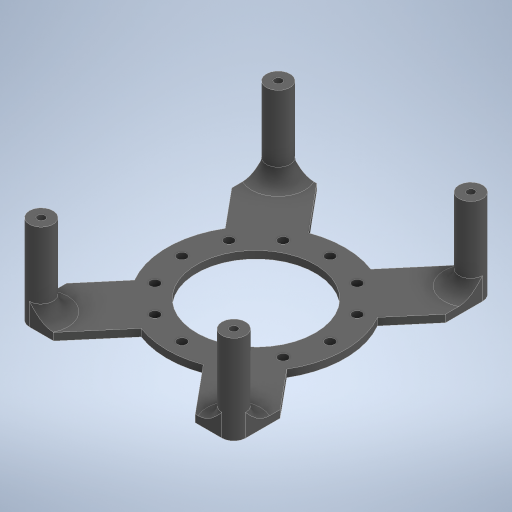
# Autodesk Inventor part: board_base_connect
Saved by Autodesk Inventor 2024.1 (Build 281209000, 209)
## iProperties
Created: 2024-08-02
Part Number: board_base_connect
Material: 一般
Document SubType Name: Modeling
Designer: hibik
Density: 1 g/cm^3
Appearance: 既定
Author: hibik
Autodesk Inventor part; units mm, degrees
ref_plane "YZ Plane" through (0, 0, 0) normal (1, 0, 0) x (0, 1, 0)
ref_plane "XZ Plane" through (0, 0, 0) normal (0, 1, 0) x (-1, 0, 0)
ref_plane "XY Plane" through (0, 0, 0) normal (0, 0, 1) x (1, 0, 0)
sketch "スケッチ1" plane through (0, 0, 0) normal (0, 1, 0) x (-1, 0, 0)
  line L0 (-32.5, -40) -> (32.5, -40) construction
  line L1 (32.5, -40) -> (32.5, 40) construction
  line L2 (32.5, 40) -> (-32.5, 40) construction
  line L3 (-32.5, 40) -> (-32.5, -40) construction
  line L4 (-32.5, -40) -> (32.5, 40) construction
  line L5 (32.5, -40) -> (-32.5, 40) construction
  circle A0 centre (32.5, 40) radius 4
  circle A1 centre (32.5, -40) radius 4
  circle A2 centre (-32.5, -40) radius 4
  circle A3 centre (-32.5, 40) radius 4
  circle A4 centre (32.5, 40) radius 1.3
  circle A5 centre (32.5, -40) radius 1.3
  circle A6 centre (-32.5, 40) radius 1.3
  circle A7 centre (-32.5, -40) radius 1.3
  point P0 (0, 0)
  dimension "d0" = 65
  dimension "d1" = 80
  dimension "d2" = 8
  dimension "d4" = 2.6
  constraints: 12 end point, 8 centre point, 8 coincident, 6 equal radius, 2 midpoint, 2 parallel, 1 horizontal, 1 perpendicular
  measures "d0" distance of L2.end L1.end
  measures "d1" distance of L1.end L0.end
  measures "d2" diameter of A0
  measures "d4" diameter of A4
extrude "押し出し1" add sketch "スケッチ1" along normal blind 30
sketch "スケッチ2" plane through (32.5, 0, 40) normal (0, -1, 0) x (1, 0, 0)
  circle A0 centre (-32.5, -40) radius 20
  circle A1 centre (-32.5, -40) radius 30
  circle A2 centre (-32.5, -15) radius 1.6
  line L0 (-32.5, -40) -> (-32.5, -10) construction
  line L1 (-32.5, -20) -> (-32.5, -10)
  circle A3 centre (-45, -18.3494) radius 1.6
  circle A4 centre (-54.1506, -27.5) radius 1.6
  circle A5 centre (-57.5, -40) radius 1.6
  circle A6 centre (-54.1506, -52.5) radius 1.6
  circle A7 centre (-45, -61.6506) radius 1.6
  circle A8 centre (-32.5, -65) radius 1.6
  circle A9 centre (-20, -61.6506) radius 1.6
  circle A10 centre (-10.8494, -52.5) radius 1.6
  circle A11 centre (-7.5, -40) radius 1.6
  circle A12 centre (-10.8494, -27.5) radius 1.6
  circle A13 centre (-20, -18.3494) radius 1.6
  line L2 (-69, 4) -> (4, 4)
  line L3 (4, 4) -> (4, -84)
  line L4 (4, -84) -> (-69, -84)
  line L5 (-69, -84) -> (-69, 4)
  circle A14 centre (0, 0) radius 4 projected
  circle A15 centre (0, -80) radius 4 projected
  circle A16 centre (-65, -80) radius 4 projected
  circle A17 centre (-65, 0) radius 4 projected
  line L6 (11.6965, -2.3846) -> (-61.3035, -90.3846)
  line L7 (-61.3035, -90.3846) -> (-76.6965, -77.6154)
  line L8 (-76.6965, -77.6154) -> (-3.6965, 10.3846)
  line L9 (-3.6965, 10.3846) -> (11.6965, -2.3846)
  line L10 (11.6965, -2.3846) -> (-76.6965, -77.6154) construction
  line L11 (-61.3035, -90.3846) -> (-3.6965, 10.3846) construction
  line L12 (-77.1651, -2.9493) -> (-3.0654, -90.0134)
  line L13 (-3.0654, -90.0134) -> (12.1651, -77.0507)
  line L14 (12.1651, -77.0507) -> (-61.9346, 10.0134)
  line L15 (-61.9346, 10.0134) -> (-77.1651, -2.9493)
  line L16 (-77.1651, -2.9493) -> (12.1651, -77.0507) construction
  line L17 (-3.0654, -90.0134) -> (-61.9346, 10.0134) construction
  point P0 (-69, 0)
  point P1 (-69, -80)
  point P2 (-65, -84)
  point P3 (0, -84)
  point P4 (4, -80)
  point P5 (4, 0)
  point P6 (0, 4)
  point P7 (-65, 4)
  point P8 (-22.1381, -11.8463)
  point P9 (-43.2167, -11.9794)
  point P10 (-56.8166, 4)
  point P11 (-69, -12.543)
  point P12 (-58.4472, -24.942)
  point P13 (-58.255, -55.3845)
  point P14 (-69, -68.3374)
  point P15 (-56.0071, -84)
  point P16 (-42.8619, -68.1537)
  point P17 (-21.7833, -68.0206)
  point P18 (-8.1834, -84)
  point P19 (4, -67.457)
  point P20 (-6.5528, -55.058)
  point P21 (-6.745, -24.6155)
  point P22 (4, -11.6626)
  point P23 (-8.9929, 4)
  dimension "d7" = 40
  dimension "d8" = 60
  dimension "d9" = 3.2
  dimension "d12" = 360
  dimension "d17" = 20
  constraints: 36 end point, 12 centre point, 6 midpoint, 6 parallel, 4 perpendicular, 4 tangent, 3 point on line, 2 coincident, 1 collinear, 1 equal length, 1 horizontal, 1 vertical, 1 vertical alignment, 30 other
  measures "d9" diameter of A2
  measures "d17" distance between parallel lines of L8 L6
extrude "押し出し2" add sketch "スケッチ2" against normal blind 2.5 contours A0 L6 A12 A1 L14 | A0 L8 A1 L6 A12 | L14 A1 L12 A0 | A0 L1 A2 A1 L8 | L12 A1 L6 A0 | L14 L3 A15 L4 L12 A1 | A0 L14 A1 L1 A2 | L8 L2 A14 L3 L6 A1 | L6 A1 L8 A6 A0 | A0 L12 A1 L14 | L8 A6 A1 L12 A0 | L6 L4 A16 L5 L8 A1 | A1 L12 L5 A17 L2 L14
fillet "フィレット1" radius 5 6 edges at (-29.6716, 2.5, -37.1716) (-29.6716, 2.5, 37.1716) (32.5, 2.5, 36) (29.6716, 2.5, 42.8284) (29.6716, 2.5, -42.8284) (32.5, 2.5, -36)
